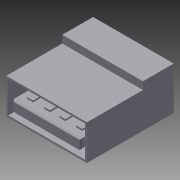
# Autodesk Inventor part: usb host con
Saved by Autodesk Inventor 2012 (Build 160160000, 160)
## iProperties
Created: 2012-02-28
Part Number: usb host con
Material: Default
Document SubType Name: Modeling
Designer: Grailas
Density: 1 g/cm^3
Author: Grailas
Autodesk Inventor part; units mm, degrees
ref_plane "YZ Plane" through (0, 0, 0) normal (1, 0, 0) x (0, 1, 0)
ref_plane "XZ Plane" through (0, 0, 0) normal (0, 1, 0) x (-1, 0, 0)
ref_plane "XY Plane" through (0, 0, 0) normal (0, 0, 1) x (1, 0, 0)
sketch "Sketch1" plane through (0, 0, 0) normal (0, 0, 1) x (1, 0, 0)
  line L0 (-6.55, 7.05) -> (6.55, 7.05)
  line L1 (6.55, 7.05) -> (6.55, -7.05)
  line L2 (6.55, -7.05) -> (-6.55, -7.05)
  line L3 (-6.55, -7.05) -> (-6.55, 7.05)
  point P0 (0, 0)
  point P1 (-6.55, 0)
  point P2 (0, 7.05)
  dimension "d0" = 13.1
  dimension "d1" = 14.1
  constraints: 8 end point, 2 midpoint, 2 parallel, 1 horizontal, 1 horizontal alignment, 1 perpendicular, 1 vertical alignment
  measures "d0" distance of L1.end L2.end
  measures "d1" distance of L0.end L1.end
extrude "Extrusion1" add sketch "Sketch1" along normal blind 5.72
sketch "Sketch2" plane through (0, 0, 5.72) normal (0, 0, 1) x (1, 0, 0)
  line L0 (6.55, 7.05) -> (6.55, -7.05) projected
  line L1 (-6.55, 7.05) -> (6.55, 7.05)
  line L2 (6.55, 7.05) -> (6.55, 2.05)
  line L3 (6.55, 2.05) -> (-6.55, 2.05)
  line L4 (-6.55, 2.05) -> (-6.55, 7.05)
  point P0 (0, 0)
  dimension "d4" = 5
  constraints: 8 end point, 2 parallel, 1 horizontal, 1 perpendicular, 1 point on line
  measures "d4" distance between parallel lines of L1 L3
extrude "Extrusion2" add sketch "Sketch2" along normal blind 1.23
sketch "Sketch3" plane through (-6.55, -7.05, 0) normal (0, -1, 0) x (1, 0, 0)
  line L0 (13.1, 5.72) -> (0, 5.72) projected
  line L1 (0, 0) -> (0, 5.72) projected
  line L2 (13.1, 0) -> (0, 0) projected
  line L3 (13.1, 0) -> (13.1, 5.72) projected
  line L4 (0.3, 5.42) -> (12.8, 5.42)
  line L5 (12.8, 5.42) -> (12.8, 0.3)
  line L6 (12.8, 0.3) -> (0.3, 0.3)
  line L7 (0.3, 0.3) -> (0.3, 5.42)
  line L8 (1, 2.86) -> (12.1, 2.86)
  line L9 (12.1, 2.86) -> (12.1, 1.02)
  line L10 (12.1, 1.02) -> (1, 1.02)
  line L11 (1, 1.02) -> (1, 2.86)
  line L12 (2.05, 2.86) -> (3.05, 2.86)
  line L13 (4.8, 2.86) -> (5.8, 2.86)
  line L14 (7.3, 2.86) -> (8.3, 2.86)
  line L15 (10.05, 2.86) -> (11.05, 2.86)
  point P0 (6.55, 0)
  dimension "d7" = 0.3
  dimension "d9" = 5.72
  dimension "d10" = 5.12
  dimension "d11" = 0.7
  dimension "d13" = 1.84
  dimension "d14" = 0.7
  dimension "d17" = 2.56
  constraints: 24 end point, 5 horizontal, 4 point on line, 2 parallel, 1 perpendicular, 3 other
  measures "d7" distance between parallel lines of L1 L7
  measures "d9" distance between parallel lines of L2 L0
  measures "d10" distance between parallel lines of L6 L4
  measures "d11" distance between parallel lines of L7 L11
  measures "d13" distance of L10.end L8.start
  measures "d14" distance between parallel lines of L5 L9
  measures "d17" distance between parallel lines of L4 L8
extrude "Extrusion3" cut sketch "Sketch3" against normal blind 10.3 contours L4 L5 L6 L7
fillet "Fillet3" radius 0.64 1 edges at (5.55, -1.9, 1.02)
fillet "Fillet4" radius 0.64 1 edges at (-5.55, -1.9, 1.02)
chamfer "Chamfer1" distance 0.2 angle 45 5 edges at (5.55, -7.05, 2.26) (5.3625, -7.05, 1.2075) (0, -7.05, 1.02) (-5.3625, -7.05, 1.2075) (-5.55, -7.05, 2.26)
chamfer "Chamfer7" distance 0.2 angle 45 1 edges at (0, -7.05, 2.86)
sketch "Sketch4" plane through (-6.55, 3.25, 0) normal (0, -1, 0) x (1, 0, 0)
  line L0 (12.1, 2.86) -> (1, 2.86) projected
  line L1 (12.1, 1.66) -> (12.1, 2.86) projected
  line L2 (2.05, 2.86) -> (3.05, 2.86)
  line L3 (3.05, 2.86) -> (3.05, 3.11)
  line L4 (3.05, 3.11) -> (2.05, 3.11)
  line L5 (2.05, 3.11) -> (2.05, 2.86)
  line L6 (4.8, 2.86) -> (5.8, 2.86)
  line L7 (5.8, 2.86) -> (5.8, 3.11)
  line L8 (5.8, 3.11) -> (4.8, 3.11)
  line L9 (4.8, 3.11) -> (4.8, 2.86)
  line L10 (7.3, 2.86) -> (8.3, 2.86)
  line L11 (8.3, 2.86) -> (8.3, 3.11)
  line L12 (8.3, 3.11) -> (7.3, 3.11)
  line L13 (7.3, 3.11) -> (7.3, 2.86)
  line L14 (10.05, 2.86) -> (11.05, 2.86)
  line L15 (11.05, 2.86) -> (11.05, 3.11)
  line L16 (11.05, 3.11) -> (10.05, 3.11)
  line L17 (10.05, 3.11) -> (10.05, 2.86)
  point P0 (6.55, 0)
  dimension "d57" = 1
  dimension "d58" = 1
  dimension "d59" = 1
  dimension "d60" = 1
  dimension "d61" = 0.25
  dimension "d62" = 0.25
  dimension "d63" = 0.25
  dimension "d64" = 0.25
  dimension "d65" = 1.5
  dimension "d66" = 1.75
  dimension "d67" = 1.75
  dimension "d68" = 1.05
  constraints: 32 end point, 8 parallel, 4 horizontal, 4 perpendicular, 4 point on line
  measures "d57" distance of L3.end L4.end
  measures "d58" distance of L7.end L8.end
  measures "d59" distance of L11.end L12.end
  measures "d60" distance of L15.end L16.end
  measures "d61" distance of L4.end L2.start
  measures "d62" distance of L8.end L6.start
  measures "d63" distance of L12.end L10.start
  measures "d64" distance of L16.end L14.start
  measures "d65" distance between parallel lines of L13 L7
  measures "d66" distance between parallel lines of L17 L11
  measures "d67" distance between parallel lines of L3 L9
  measures "d68" distance between parallel lines of L1 L15
extrude "Extrusion5" add sketch "Sketch4" along normal blind 9
body "Solid1"
